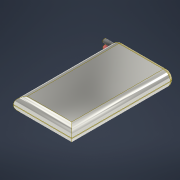
# Autodesk Inventor part: 600mah Battery
Saved by Autodesk Inventor 2022 (Build 260153000, 153)
## iProperties
Created: 2021-04-24
Part Number: 600mah Battery
Material: Generic
Document SubType Name: Modeling
Designer: sidsa
Density: 1 g/cm^3
Appearance: Silver
Author: sidsa
Autodesk Inventor part; units mm, degrees
ref_plane "YZ Plane" through (0, 0, 0) normal (1, 0, 0) x (0, 1, 0)
ref_plane "XZ Plane" through (0, 0, 0) normal (0, 1, 0) x (-1, 0, 0)
ref_plane "XY Plane" through (0, 0, 0) normal (0, 0, 1) x (1, 0, 0)
sketch "Sketch1" plane through (0, 0, 0) normal (0, 1, 0) x (-1, 0, 0)
  line L0 (0, 0) -> (25.4, 0)
  line L1 (25.4, 0) -> (25.4, -44.45)
  line L2 (25.4, -44.45) -> (0, -44.45)
  line L3 (0, -44.45) -> (0, 0)
  dimension "d0" = 25.4
  dimension "d1" = 44.45
  constraints: 8 end point, 2 parallel, 1 horizontal, 1 perpendicular
  measures "d0" distance of L1.end L2.end
  measures "d1" distance of L2.end L0.start
extrude "Extrusion1" add sketch "Sketch1" along normal blind 6.35
fillet "Fillet1" radius 3.048 6 edges at (0, 6.35, -22.225) (0, 0, -22.225) (-12.7, 0, 0) (-12.7, 6.35, 0) (-25.4, 6.35, -22.225) (-25.4, 0, -22.225)
fillet "Fillet2" radius 1.5875 4 edges at (-24.5073, 5.4573, -44.45) (-12.7, 0, -44.45) (-0.8927, 5.4573, -44.45) (-12.7, 6.35, -44.45)
sketch "Sketch2" plane through (-25.4, 3.048, -42.8625) normal (-1, 0, 0) x (0, 0, 1)
  line L0 (0, 0.254) -> (0, 0) projected
  line L1 (0, 0.127) -> (2.6469, 0.127)
  circle A0 centre (0, 1.3103) radius 0.7937
  circle A1 centre (0, -1.0563) radius 0.7937
  point P0 (42.8625, -3.048)
  dimension "d6" = 1.5875
  constraints: 2 centre point, 2 end point, 1 horizontal, 1 midpoint, 1 symmetric about line, 1 other
  measures "d6" diameter of A0
extrude "Extrusion2" add sketch "Sketch2" along normal mid plane 6.35
body "Solid1"
